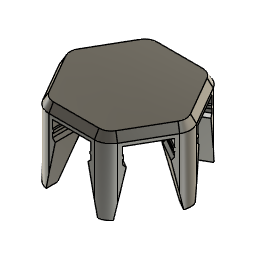
RegularNode (Autodesk Fusion 360 design; units mm, degrees)
Autodesk Fusion 360 part; units mm, degrees
sketch "Sketch1" plane through (0, 0, 0) normal (0, 0, 1) x (1, 0, 0)
  line L0 (28.8675, 0) -> (14.4338, 25)
  line L1 (14.4338, 25) -> (-14.4338, 25)
  line L2 (-14.4338, 25) -> (-28.8675, 0)
  line L3 (-28.8675, 0) -> (-14.4338, -25)
  line L4 (-14.4338, -25) -> (14.4338, -25)
  line L5 (14.4338, -25) -> (28.8675, 0)
  dimension "d1" = 25
  constraint horizontal L1
  measures "d1" distance of origin L5
extrude "Extrude1" add sketch "Sketch1" along normal blind 5
extrude "Extrude2" add sketch "Sketch1" against normal blind 28
sketch "Sketch2" plane through (0, 25, 0) normal (0, 1, 0) x (-1, 0, 0)
  line L0 (14.4338, -28) -> (14.4338, 5)
  line L1 (14.4338, 5) -> (-14.4338, 5)
  line L2 (-14.4338, 5) -> (-14.4338, -28)
  line L3 (-14.4338, -28) -> (14.4338, -28)
  line L4 (0, 5) -> (0, -28)
  line L5 (-14.4338, 0) -> (14.4338, 0)
  line L6 (-8.5, 0) -> (-8.5, -3.5)
  line L7 (-8.5, -3.5) -> (-8.1, -3.9)
  line L8 (-8.1, -3.9) -> (-8.1, -5.1)
  line L9 (-8.1, -5.1) -> (-8.5, -5.1)
  line L10 (-8.5, -5.1) -> (-8.5, -7)
  line L11 (-8.5, -7) -> (-7.3, -8.2)
  line L12 (-7.3, -8.2) -> (-11.4338, -28)
  line L13 (8.5, -3.5) -> (8.1, -3.9)
  line L14 (8.1, -3.9) -> (8.1, -5.1)
  line L15 (8.1, -5.1) -> (8.5, -5.1)
  line L16 (8.5, -5.1) -> (8.5, -7)
  line L17 (8.5, -7) -> (7.3, -8.2)
  line L18 (7.3, -8.2) -> (11.4338, -28)
  line L19 (8.5, 0) -> (8.5, -3.5)
  line L20 (0, -0.8) -> (-6.25, -0.8)
  line L21 (-6.25, -0.8) -> (-6.25, -1.3523)
  line L22 (-6.25, -1.3523) -> (-6.25, -3.1707)
  line L23 (-7.3, -8.2) -> (-6.25, -3.1707)
  line L24 (6.25, -0.8) -> (6.25, -1.3523)
  line L25 (6.25, -1.3523) -> (6.25, -3.1707)
  line L26 (7.3, -8.2) -> (6.25, -3.1707)
  line L27 (0, -0.8) -> (6.25, -0.8)
  dimension "d6" = 17
  dimension "d7" = 135
  dimension "d8" = 3.5
  dimension "d9" = 0.4
  dimension "d10" = 1.2
  dimension "d11" = 135
  dimension "d12" = 1.2
  dimension "d13" = 7
  dimension "d17" = 0.8
  dimension "d19" = 2.25
  dimension "d29" = 3
  constraint midpoint L1 L4.start
  constraint midpoint L3 L4.end
  constraint coincident L5 L6.start
  constraint perpendicular L5 L6
  constraint perpendicular L5 L8
  constraint perpendicular L8 L9
  constraint perpendicular L3 L10
  constraint coincident L3 L12.end
  constraint symmetric L4 L6.start L19.start
  constraint symmetric L4 L6.end L13.start
  constraint symmetric L4 L7.end L13.end
  constraint symmetric L4 L8.end L14.end
  constraint symmetric L4 L9.end L15.end
  constraint symmetric L4 L10.end L16.end
  constraint symmetric L4 L11.end L17.end
  constraint symmetric L4 L12.end L18.end
  constraint collinear L6 L10
  constraint coincident L4 L20.start
  constraint perpendicular L4 L20
  constraint perpendicular L20 L21
  constraint perpendicular L20 L22
  constraint collinear L12 L23
  constraint symmetric L4 L20.start L27.start
  constraint symmetric L4 L20.end L24.start
  constraint symmetric L4 L21.end L24.end
  constraint symmetric L4 L22.end L25.end
  measures "d6" distance of L6 L19
  measures "d7" angle of L6 L7
  measures "d8" distance of L6.start L6.end
  measures "d9" horizontal distance of L6.end L7.end
  measures "d10" distance of L7.end L8.end
  measures "d11" angle of L10 L11
  measures "d12" horizontal distance of L10.end L11.end
  measures "d13" distance of L6.start L10.end
  measures "d17" distance of L5 L20
  measures "d19" distance of L6 L22
  measures "d29" distance of L0.start L18.end
extrude "Extrude3" cut sketch "Sketch2" against normal blind 10 contours L3 L4 L18 L24 L25 L26 L27 | L4 L5 L13 L14 L15 L16 L17 L19 L24 L25 L26 L27 | L3 L4 L12 L20 L21 L22 L23 | L4 L5 L6 L7 L8 L9 L10 L11 L20 L21 L22 L23
extrude "Extrude4" cut sketch "Sketch2" against normal blind 27 contours L3 L4 L18 L24 L25 L26 L27 | L3 L4 L12 L20 L21 L22 L23
pattern_circular "C-Pattern1" count 6 over 360 about axis through (0, 0, -46.5) along (0, 0, 1) of "Extrude3", "Extrude4"
fillet "Fillet2" radius 7.5 6 edges at (-28.8675, 0, -11.5) (-14.4338, 25, -11.5) (-14.4338, -25, -11.5) (14.4338, -25, -11.5) (28.8675, 0, -11.5) (14.4338, 25, -11.5)
chamfer "Chamfer1" distance 2 angle 60 12 edges at (21.6506, -12.5, 5) (27.7073, 0, 5) (21.6506, 12.5, 5) (13.8536, 23.9952, 5) (0, 25, 5) (-13.8536, 23.9952, 5) (-21.6506, 12.5, 5) (-27.7073, 0, 5) (-21.6506, -12.5, 5) (-13.8536, -23.9952, 5) (0, -25, 5) (13.8536, -23.9952, 5) measured on face at (6.7358, 2.5, 5) measured on face at (27.3392, -2.3205, -6) measured on face at (6.7358, 2.5, 5) measured on face at (15.6793, 22.5162, -6) measured on face at (6.7358, 2.5, 5) measured on face at (-11.66, 24.8367, -6) measured on face at (6.7358, 2.5, 5) measured on face at (-27.3392, 2.3205, -6) measured on face at (6.7358, 2.5, 5) measured on face at (-15.6793, -22.5162, -6) measured on face at (6.7358, 2.5, 5) measured on face at (15.6793, -22.5162, -6)
fillet "Fillet1" [rolled back] radius 1.5
mirror "Mirror1" [rolled back] mirror stitch tolerance 0.1
ref_plane "WorkPlane1" through (13.0705, -17.3612, -1.75) normal (0.5, 0.866025, 0) x (0, 0, -1)
ref_plane "WorkPlane2" through (-13.0705, -17.3612, -1.75) normal (-0.5, 0.866025, 0) x (0, 0, 1)
split "Split1" [suppressed]
split "Split2" [suppressed]
equation "d4 = -( 20 mm + 8 mm )"
